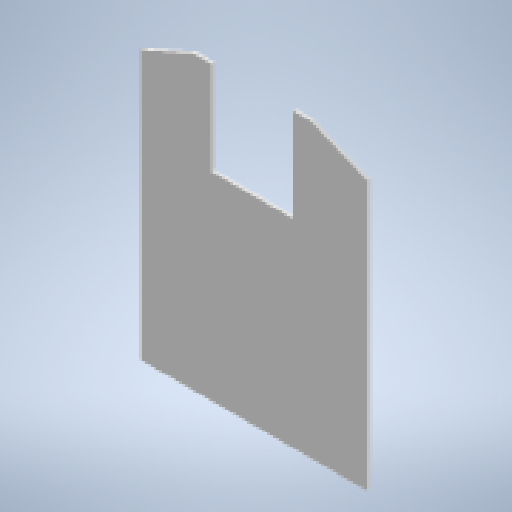
# Autodesk Inventor part: car platform
Saved by Autodesk Inventor 2023.2 (Build 272271030, 271C)
## iProperties
Created: 2023-06-19
Part Number: car platform
Material: Generic
Document SubType Name: Modeling
Designer: kao91
Density: 1 g/cm^3
Appearance: Default
Author: kao91
Autodesk Inventor part; units mm, degrees
ref_plane "YZ Plane" through (0, 0, 0) normal (1, 0, 0) x (0, 1, 0)
ref_plane "XZ Plane" through (0, 0, 0) normal (0, 1, 0) x (-1, 0, 0)
ref_plane "XY Plane" through (0, 0, 0) normal (0, 0, 1) x (1, 0, 0)
sketch "Sketch1" plane through (0, 0, 0) normal (0, 0, 1) x (1, 0, 0)
  line L0 (151.725, 24) -> (151.725, -206)
  line L1 (151.725, -206) -> (-41.7, -206)
  line L2 (-41.7, -206) -> (-41.7, 24)
  line L3 (151.725, 24) -> (103.3, 44)
  line L4 (3.3, 44) -> (-41.7, 24)
  line L5 (78.3, 44) -> (78.3, -16)
  line L6 (3.3, 44) -> (18.3, 44)
  line L7 (78.3, 44) -> (103.3, 44)
  line L8 (-34.2, -33.5) -> (-34.2, 11.5) projected
  line L9 (-2.95, 11.5) -> (-2.95, -33.5) projected
  line L10 (-36.7, -41) -> (-0.45, -41)
  line L11 (-0.45, -41) -> (-0.45, 19)
  line L12 (-0.45, 19) -> (-36.7, 19)
  line L13 (-36.7, 19) -> (-36.7, -41)
  line L14 (110.475, -41) -> (146.725, -41)
  line L15 (146.725, -41) -> (146.725, 19)
  line L16 (146.725, 19) -> (110.475, 19)
  line L17 (110.475, 19) -> (110.475, -41)
  line L18 (110.475, -191) -> (146.725, -191)
  line L19 (146.725, -191) -> (146.725, -131)
  line L20 (146.725, -131) -> (110.475, -131)
  line L21 (110.475, -131) -> (110.475, -191)
  line L22 (-36.7, -191) -> (-0.45, -191)
  line L23 (-0.45, -191) -> (-0.45, -131)
  line L24 (-0.45, -131) -> (-36.7, -131)
  line L25 (-36.7, -131) -> (-36.7, -191)
  line L26 (144.225, -33.5) -> (144.225, 11.5) projected
  line L27 (112.975, 11.5) -> (112.975, -33.5) projected
  line L28 (112.975, -183.5) -> (112.975, -138.5) projected
  line L29 (144.225, -138.5) -> (144.225, -183.5) projected
  line L30 (-34.2, -138.5) -> (-34.2, -183.5) projected
  line L31 (-2.95, -183.5) -> (-2.95, -138.5) projected
  line L32 (75.3, -16) -> (75.2995, -26)
  line L33 (75.2995, -26) -> (78.2995, -26)
  line L34 (78.2995, -26) -> (78.3, -16)
  line L35 (65.3, -16) -> (65.2995, -26)
  line L36 (65.2995, -26) -> (68.2995, -26)
  line L37 (68.2995, -26) -> (68.3, -16)
  line L38 (55.3, -16) -> (55.2995, -26.1226)
  line L39 (55.2995, -26.1226) -> (58.2995, -26.1227)
  line L40 (58.2995, -26.1227) -> (58.3, -16)
  line L41 (78.3, -16) -> (78.3, -16)
  line L42 (75.3, -16) -> (68.3, -16)
  line L43 (65.3, -16) -> (58.3, -16)
  line L44 (45.3, -16) -> (45.2995, -25.9999)
  line L45 (48.2995, -26) -> (48.3, -16)
  line L46 (45.2995, -25.9999) -> (48.2995, -26)
  line L47 (55.3, -16) -> (48.3, -16)
  line L48 (38.2995, -26) -> (38.3, -16)
  line L49 (35.2995, -26) -> (38.2995, -26)
  line L50 (35.3, -16) -> (35.2995, -26)
  line L51 (28.2995, -26) -> (28.3, -16)
  line L52 (25.2995, -26) -> (28.2995, -26)
  line L53 (25.3, -16) -> (25.2995, -26)
  line L54 (45.3, -16) -> (38.3, -16)
  line L55 (35.3, -16) -> (28.3, -16)
  line L56 (18.3, 44) -> (25.3, 44)
  line L57 (25.3, 44) -> (25.3, -16)
  point P0 (-34.2, -11)
  point P1 (-36.7, -11)
  point P2 (128.6, -41)
  point P3 (110.475, -11)
  point P4 (112.975, -11)
  point P5 (128.6, -191)
  point P6 (128.6, -131)
  point P7 (110.475, -161)
  point P8 (112.975, -161)
  point P9 (-36.7, -161)
  point P10 (-34.2, -161)
  point P11 (75.2998, -21)
  point P12 (78.2998, -21)
  point P13 (76.775, -16.5)
  point P14 (76.7995, -26)
  point P15 (65.2998, -21)
  point P16 (68.2998, -21)
  point P17 (66.775, -16.5)
  point P18 (66.7995, -26)
  point P19 (55.2998, -21.0613)
  point P20 (58.2998, -21.0613)
  point P21 (56.775, -16.5)
  point P22 (56.7995, -26.1226)
  point P23 (45.2998, -20.9999)
  point P24 (46.7995, -25.9999)
  point P25 (43.0984, -16.3775)
  point P26 (48.2998, -21)
  point P27 (38.2998, -21)
  point P28 (36.7995, -26)
  point P29 (35.2998, -21)
  point P30 (28.2998, -21)
  point P31 (26.7995, -26)
  point P32 (25.2998, -21)
  point P33 (21.8, -16)
  point P34 (78.3, -16)
  point P35 (51.8, -16)
  point P36 (71.8, -16)
  dimension "d19" = 20
  dimension "d21" = 20
  dimension "d23" = 100
  dimension "d26" = 60
  dimension "d29" = 250
  dimension "d32" = 2.5
  dimension "d33" = 2.5
  dimension "d34" = 60
  dimension "d35" = 0
  dimension "d36" = 5
  dimension "d37" = 25
  dimension "d39" = 2.5
  dimension "d40" = 2.5
  dimension "d41" = 5
  dimension "d43" = 60
  dimension "d44" = 0
  dimension "d45" = 60
  dimension "d46" = 2.5
  dimension "d47" = 0
  dimension "d48" = 2.5
  dimension "d49" = 2.5
  dimension "d50" = 2.5
  dimension "d51" = 60
  dimension "d52" = 0
  dimension "d55" = 250
  dimension "d75" = 3
  dimension "d76" = 10
  dimension "d77" = 7
  dimension "d79" = 3
  dimension "d80" = 10
  dimension "d81" = 3
  dimension "d82" = 10
  dimension "d84" = 7
  dimension "d86" = 7
  dimension "d87" = 7
  dimension "d88" = 3
  dimension "d89" = 3
  dimension "d90" = 3
  dimension "d92" = 7
  dimension "d93" = 45
  dimension "d95" = 90
  dimension "d98" = 10
  dimension "d100" = 10
  dimension "d101" = 10
  dimension "d102" = 10
  dimension "d103" = 60
  dimension "d104" = 60
  dimension "d105" = 60
  dimension "d106" = 60
  dimension "d108" = 0
  dimension "d112" = 22
  dimension "d113" = 53
  constraints: 100 end point, 32 midpoint, 17 parallel, 6 horizontal, 6 perpendicular, 2 point on line
  measures "d19" vertical distance of L3.end L0.start
  measures "d21" vertical distance of L4.start L2.end
  measures "d23" distance of L3.end L4.start
  measures "d26" distance of L5.start L5.end
  measures "d29" vertical distance of L1.end L4.start
  measures "d32" distance between parallel lines of L11 L9
  measures "d33" distance between parallel lines of L13 L8
  measures "d34" distance between parallel lines of L12 L10
  measures "d35" vertical distance of point (-34.2, -11) point (-36.7, -11)
  measures "d36" distance between parallel lines of L2 L13
  measures "d37" vertical distance of L11.end L4.start
  measures "d39" distance between parallel lines of L17 L27
  measures "d40" distance between parallel lines of L15 L26
  measures "d41" distance between parallel lines of L0 L15
  measures "d43" distance from line of point (128.6, -41) L16
  measures "d44" vertical distance of point (110.475, -11) point (112.975, -11)
  measures "d45" distance of point (128.6, -191) point (128.6, -131)
  measures "d46" distance between parallel lines of L28 L21
  measures "d47" vertical distance of point (110.475, -161) point (112.975, -161)
  measures "d48" distance between parallel lines of L19 L29
  measures "d49" distance between parallel lines of L30 L25
  measures "d50" distance between parallel lines of L23 L31
  measures "d51" distance between parallel lines of L22 L24
  measures "d52" vertical distance of point (-36.7, -161) point (-34.2, -161)
  measures "d55" vertical distance of L3.end L0.end
  measures "d75" distance of L46.start L45.start
  measures "d76" distance of L45.end L45.start
  measures "d77" distance between parallel lines of L45 L38
  measures "d79" distance of L49.start L49.end
  measures "d80" distance of L48.end L49.end
  measures "d81" distance of L52.start L52.end
  measures "d82" distance of L51.end L52.end
  measures "d84" distance between parallel lines of L48 L44
  measures "d86" distance between parallel lines of L37 L32
  measures "d87" distance between parallel lines of L40 L35
  measures "d88" distance of L32.end L33.end
  measures "d89" distance of L35.end L37.start
  measures "d90" distance of L38.end L40.start
  measures "d92" distance between parallel lines of L50 L51
  measures "d93" horizontal distance of L4.start L2.end
  measures "d95" angle of L5 L7
  measures "d98" distance of L53.start L52.start
  measures "d100" distance from line of point (78.3, -16) L33
  measures "d101" distance between parallel lines of L33 L42
  measures "d102" distance between parallel lines of L43 L36
  measures "d103" distance from line of L7 point (51.8, -16)
  measures "d104" distance from line of L7 point (71.8, -16)
  measures "d105" distance between parallel lines of L43 L7
  measures "d106" distance from line of L6.end L47
  measures "d108" distance of L34.end L5.end
  measures "d112" distance of L4.start L56.end
  measures "d113" distance between parallel lines of L5 L57
extrude "Extrusion2" add sketch "Sketch1" along normal blind 3
body "Solid2"
